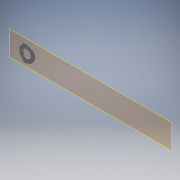
# Autodesk Inventor part: Encoder Mount
Saved by Autodesk Inventor 2016 (Build 200138000, 138)
## iProperties
Created: 2017-01-21
Part Number: Encoder Mount
Material: Generic
Document SubType Name: Modeling
Designer: Moonlight.Admin
Density: 1 g/cm^3
Appearance: Default
Author: Moonlight.Admin
Autodesk Inventor part; units mm, degrees
ref_plane "YZ Plane" through (0, 0, 0) normal (1, 0, 0) x (0, 1, 0)
ref_plane "XZ Plane" through (0, 0, 0) normal (0, 1, 0) x (-1, 0, 0)
ref_plane "Work Plane1" through (0, 0, 0) normal (0, 0, 1) x (1, 0, 0)
sketch "Sketch1" plane through (0, 0, 0) normal (0, 0, 1) x (1, 0, 0)
  line L0 (38.5336, 66.2269) -> (46.4641, 63.2899)
  line L1 (63.0428, 39.4709) -> (63.0428, 36.7291)
  line L2 (46.4641, 12.9101) -> (38.5336, 9.9731)
  line L3 (24.0727, 14.1184) -> (17.5423, 22.5716)
  line L4 (17.5423, 53.6284) -> (24.0727, 62.0816)
  circle A0 centre (37.6428, 38.1) radius 14.2875 projected
  circle A1 centre (32.8676, 57.15) radius 2.0193 projected
  circle A2 centre (32.8676, 19.05) radius 2.0193 projected
  line L5 (37.6428, 38.1) -> (32.8676, 57.15) construction
  line L6 (37.6428, 38.1) -> (32.8676, 19.05) construction
  arc A3 (38.5336, 66.2269) -> (24.0727, 62.0816) centre (34.123, 54.3174) ccw
  arc A4 (24.0727, 14.1184) -> (38.5336, 9.9731) centre (34.123, 21.8826) ccw
  arc A5 (17.5423, 53.6284) -> (17.5423, 22.5716) centre (37.6428, 38.1) ccw
  arc A6 (46.4641, 12.9101) -> (63.0428, 36.7291) centre (37.6428, 36.7291) ccw
  arc A7 (63.0428, 39.4709) -> (46.4641, 63.2899) centre (37.6428, 39.4709) ccw
  line L7 (12.2428, 46.8808) -> (12.2428, 25.1015) construction
  point P0 (29.7797, 69.4689)
  point P1 (63.0428, 57.15)
  point P2 (63.0428, 19.05)
  point P3 (29.7797, 6.7311)
  point P4 (5.5461, 38.1)
  point P5 (63.0428, 38.1)
  dimension "d2" = 12.7
  dimension "d3" = 12.7
  dimension "d5" = 25.4
  dimension "d6" = 38.1
  dimension "d7" = 12.7
  dimension "d8" = 25.4
  dimension "d9" = 25.4
  constraints: 16 end point, 12 point on line, 11 tangent, 10 point on circle, 5 centre point, 2 horizontal alignment, 2 vertical, 1 equal radius, 1 midpoint
  measures "d2" distance of L5.end point (29.78, 69.469)
  measures "d3" distance of L6.end point (29.78, 6.731)
  measures "d5" distance from line of L1 L5.start
  measures "d6" distance of point (63.043, 57.15) point (63.043, 19.05)
  measures "d7" radius of A3
  measures "d8" radius of A5
  measures "d9" distance from line of L5.start L7
ref_plane "Work Plane2" through (21.5824, 22.0396, 3.2283) normal (0, 0, 1) x (0.9852, -0.1712, 0)
extrude "Extrusion1" add sketch "Sketch1" along normal up to surface (3.2283 mm away)
equation "\"d3\" = d2"
equation "\"d9\" = d5"
body "Solid1"
